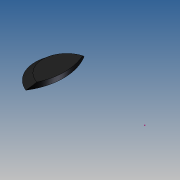
# Autodesk Inventor part: gornji shiny dio
Saved by Autodesk Inventor 2012 (Build 160160000, 160)
## iProperties
Created: 2011-11-30
Part Number: gornji shiny dio
Material: Default
Document SubType Name: Modeling
Designer: slazh bliskovic
Density: 1 g/cm^3
Mass: 4.94251 g
Surface Area: 46.167 cm^2
Volume: 4.94251 cm^3
Author: slazh bliskovic
Autodesk Inventor part; units mm, degrees
ref_plane "YZ Plane" through (0, 0, 0) normal (1, 0, 0) x (0, 1, 0)
sketch "Sketch1" plane through (0, 0, 0) normal (0, 0, 1) x (1, 0, 0)
  spline S0 degree 3 poles (12.775809, 13.743738) (13.453575, 14.296004) (14.16507, 14.792978) (16.937316, 16.441783) (19.224317, 17.243595) (24.595739, 17.979132) (27.723679, 17.596307) (32.869411, 15.535143) (34.964738, 14.129672) (38.628289, 10.359381) (40.089591, 7.896643) (41.435431, 3.545039) (41.703305, 1.772836) (41.703303, -0.000028) (41.7033, -1.772892) (41.435423, -3.545074) (40.089464, -7.897041) (38.627791, -10.360188) (34.965482, -14.128645) (32.872746, -15.532844) (27.722529, -17.597958) (24.586064, -17.980815) (19.219795, -17.240648) (16.945007, -16.443301) (14.175916, -14.800553) (13.458713, -14.300191) (12.775809, -13.743738) knots 0.0475769 0.0475769 0.0475769 0.0475769 0.30841807 0.30841807 1.01543689 1.01543689 1.92782472 1.92782472 2.66674079 2.66674079 3.49744633 3.49744633 4.02653047 4.02653047 4.02653047 4.55561461 4.55561461 5.38644202 5.38644202 6.12460097 6.12460097 7.03935565 7.03935565 7.74266001 7.74266001 8.00547976 8.00547976 8.00547976 8.00547976 weights 1 1 1 1 1 1 1 1 1 1 1 1 1 1 1 1 1 1 1 1 1 1 1 1 1 1 1
  spline S1 degree 3 poles (12.775809, -13.743738) (12.326511, -13.377635) (11.821873, -13.079408) (10.656846, -12.620046) (9.984673, -12.49013) (9.311785, -12.49013) knots 0 0 0 0 0.46270736 0.46270736 1 1 1 1 weights 1 1 1 1 1 1
  line L0 (9.311785, -12.49013) -> (-31.025337, -12.49013)
  spline S2 degree 3 poles (-31.025337, -12.49013) (-32.110865, -12.49013) (-33.198033, -12.347386) (-34.736089, -11.936981) (-35.218379, -11.77627) (-35.690276, -11.586272) knots 0 0 0 0 0.68100487 0.68100487 1 1 1 1 weights 1 1 1 1 1 1
  spline S3 degree 3 poles (9.311785, 12.49013) (9.7991, 12.49013) (10.286231, 12.55778) (11.492025, 12.895964) (12.182584, 13.260359) (12.775809, 13.743738) knots 0 0 0 0 0.38911359 0.38911359 1 1 1 1 weights 1 1 1 1 1 1
  line L1 (0, 0) -> (-42.287334, 0) construction
  line L2 (9.311785, 12.49013) -> (-31.025337, 12.49013)
  arc A0 (-31.025337, 12.49013) -> (-31.025337, -12.49013) centre (-31.025337, 0) ccw
  constraints: 2 end point, 2 point on circle, 1 centre point, 1 parallel, 1 point on line, 1 symmetric about line
sketch "Sketch1 outline for Extrusion1" plane through (0, 0, 0) normal (0, 0, 1) x (1, 0, 0)
  spline S0 degree 3 poles (12.775809, 13.743738) (13.453575, 14.296004) (14.16507, 14.792978) (16.937316, 16.441783) (19.224317, 17.243595) (24.595739, 17.979132) (27.723679, 17.596307) (32.869411, 15.535143) (34.964738, 14.129672) (38.628289, 10.359381) (40.089591, 7.896643) (41.435431, 3.545039) (41.703305, 1.772836) (41.703303, -0.000028) (41.7033, -1.772892) (41.435423, -3.545074) (40.089464, -7.897041) (38.627791, -10.360188) (34.965482, -14.128645) (32.872746, -15.532844) (27.722529, -17.597958) (24.586064, -17.980815) (19.219795, -17.240648) (16.945007, -16.443301) (14.175916, -14.800553) (13.458713, -14.300191) (12.775809, -13.743738) knots 0 0 0 0 0.03277763 0.03277763 0.12162249 0.12162249 0.23627429 0.23627429 0.3291274 0.3291274 0.4335149 0.4335149 0.50000027 0.50000027 0.50000027 0.56648564 0.56648564 0.67088845 0.67088845 0.76364643 0.76364643 0.87859564 0.87859564 0.96697374 0.96697374 1 1 1 1
  spline S1 degree 3 poles (12.775809, -13.743738) (12.326511, -13.377635) (11.821873, -13.079408) (10.656846, -12.620046) (9.984673, -12.49013) (9.311785, -12.49013) knots 0 0 0 0 0.46270736 0.46270736 1 1 1 1
  line L0 (9.311785, -12.49013) -> (-31.025337, -12.49013)
  arc A0 (-31.025337, -12.49013) -> (-31.025337, 12.49013) centre (-31.025337, 0) cw
  line L1 (-31.025337, 12.49013) -> (9.311785, 12.49013)
  spline S2 degree 3 poles (9.311785, 12.49013) (9.7991, 12.49013) (10.286231, 12.55778) (11.492025, 12.895964) (12.182584, 13.260359) (12.775809, 13.743738) knots 0 0 0 0 0.38911359 0.38911359 1 1 1 1
extrude "Extrusion1" add sketch "Sketch1 outline for Extrusion1" along normal blind 2.5
sketch "Sketch6" plane through (0, 0, 2.5) normal (0, 0, 1) x (1, 0, 0)
  line L0 (-9.525285, -2.542488) -> (-15.356425, -2.542488) construction
  line L1 (-15.356425, -2.542488) -> (-15.356425, 2.542488) construction
  line L2 (-15.356425, 2.542488) -> (-9.525285, 2.542488) construction
  line L3 (-9.525285, 2.542488) -> (-9.525285, -2.542488) construction
  point P0 (0, 0)
  point P1 (-6.22634, 0)
  constraints: 1 horizontal alignment, 2 other
decal "Decal1"
ref_plane "Work Plane1" through (0, 0, 0) normal (0.2164396, 0, 0.976296) x (0, 1, 0)
sketch "Sketch7" plane through (0, 0, 0) normal (0.2164396, 0, 0.976296) x (0, 1, 0)
  point P0 (0, 0)
ref_plane "Work Plane2" through (0, 0, 0) normal (0.2164396, 0, 0.976296) x (0, 1, 0)
sketch "Sketch8" plane through (0, 0, 0) normal (0.2164396, 0, 0.976296) x (0, 1, 0)
  spline S0 degree 3 poles (-12.778059, 35.623375) (-13.1078, 34.920563) (-13.375951, 34.191997) (-13.894146, 32.296016) (-14.054771, 31.101656) (-14.054771, 29.909099) knots -12.94996087 -12.94996087 -12.94996087 -12.94996087 -12.73961425 -12.73961425 -12.41484583 -12.41484583 -12.41484583 -12.41484583 weights 1 1 1 1 1 1
  arc A0 (-15.649435, 38.017312) -> (14.955462, 37.360965) centre (0, 53.868836) ccw
  point P0 (0, 0)
  dimension "d51" = 22.275
  constraints: 2 point on circle, 1 centre point
  measures "d51" radius of A0
surface extrude "ExtrusionSrf1" sketch "Sketch8" against normal blind 38.75 shown no curves A0
split body "Split1" result one side removed by surface "ExtrusionSrf1" removed pieces at (-4.595575, -0.488214, 0.5)
draft "FaceDraft1" angle 50 pull direction (0, 0, 1) faces at (-36.333978, 11.305825, 1.666667) fixed edges at (-43.515467, 0, 0)
body "Solid1"
body "Srf1"
